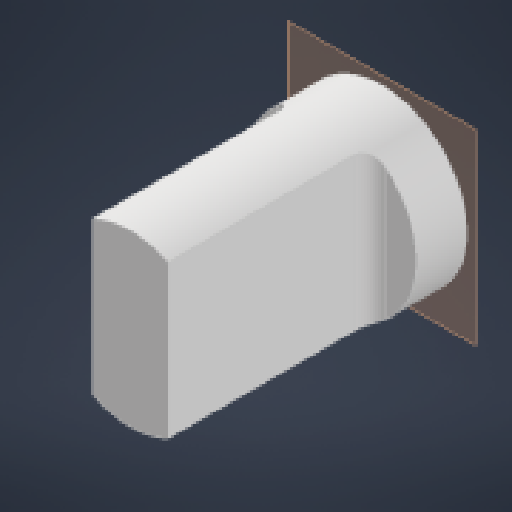
# Autodesk Inventor part: Ring
Saved by Autodesk Inventor 2025 (Build 290162000, 162)
## iProperties
Created: 2024-05-27
Part Number: Ring
Material: Generic
Document SubType Name: Modeling
Designer: zulet
Density: 1 g/cm^3
Appearance: Default
Author: zulet
Autodesk Inventor part; units mm, degrees
ref_plane "YZ Plane" through (0, 0, 0) normal (1, 0, 0) x (0, 1, 0)
ref_plane "XZ Plane" through (0, 0, 0) normal (0, 1, 0) x (-1, 0, 0)
ref_plane "XY Plane" through (0, 0, 0) normal (0, 0, 1) x (1, 0, 0)
sketch "Sketch1" plane through (0, 0, 0) normal (0, 0, 1) x (1, 0, 0)
  circle A0 centre (0, -8.4587) radius 16.9175 projected
  line L0 (7.5, -33.8588) -> (-7.5, -33.8588)
  line L1 (-7.5, -33.8588) -> (-7.5, 16.9413)
  line L2 (-7.5, 16.9413) -> (7.5, 16.9413)
  line L3 (7.5, 16.9413) -> (7.5, -33.8588)
  line L4 (7.5, -33.8588) -> (-7.5, 16.9413) construction
  line L5 (-7.5, -33.8588) -> (7.5, 16.9413) construction
  point P0 (0, 0)
  point P1 (7.5, 6.7054)
  point P2 (7.5, -23.6229)
  point P3 (-7.5, -23.6229)
  point P4 (-7.5, 6.7054)
  dimension "d0" = 15
  dimension "d1" = 50.8
  constraints: 12 end point, 2 midpoint, 2 parallel, 1 horizontal, 1 perpendicular
  measures "d0" distance of L1.end L2.end
  measures "d1" distance of L0.end L1.end
extrude "Extrusion1" add sketch "Sketch1" along normal blind 10 contours A0 L3 | L1 A0
ref_plane "Work Plane1" through (0, 0, 0) normal (0, 0, 1) x (1, 0, 0)
sketch "Sketch2" plane through (0, 0, 0) normal (0, 0, 1) x (1, 0, 0)
  circle A0 centre (0, -8.4587) radius 16.9175 projected
  line L0 (-7.5, -23.6229) -> (-7.5, 6.7054) projected
  line L1 (7.5, 6.7054) -> (7.5, -23.6229) projected
  point P0 (0, 0)
extrude "Extrusion2" add sketch "Sketch2" along normal blind 50 contours L1 A0 L0
fillet "Fillet1" radius 3.175 2 edges at (-7.5, -8.4587, 10) (7.5, -8.4587, 10)
sketch "Sketch3" plane through (-7.5, -23.6229, 50) normal (-1, 0, 0) x (0, 0, 1)
  line L0 (0, 0) -> (0, 30.3283) projected
  circle A0 centre (0, 15.1642) radius 12.5
  circle A1 centre (0, 15.1642) radius 20
  point P0 (-50, 23.6229)
  point P1 (0, 27.6642)
  point P2 (0, 2.6642)
  dimension "d7" = 25
  dimension "d8" = 40
  constraints: 2 centre point, 1 coincident, 1 midpoint
  measures "d7" diameter of A0
  measures "d8" diameter of A1
extrude "Extrusion3" add sketch "Sketch3" against normal up to surface (15 mm away)
extrude "Extrusion4" cut sketch "Sketch3" against normal through all contours A0 L0 picked at (-2.763, 18.283)
fillet "Fillet2" radius 3.175 2 edges at (-7.5, -8.4588, 70) (7.5, -8.4588, 70)
body "Solid1"
